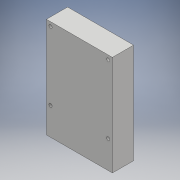
# Autodesk Inventor part: RaspberryPi_Placeholder
Saved by Autodesk Inventor 2017 (Build 210142000, 142)
## iProperties
Created: 2017-02-02
Part Number: RaspberryPi_Placeholder
Material: Generic
Document SubType Name: Modeling
Designer: Alexander Miller
Density: 1 g/cm^3
Appearance: Default
Author: Alexander Miller
Autodesk Inventor part; units mm, degrees
ref_plane "YZ Plane" through (0, 0, 0) normal (1, 0, 0) x (0, 1, 0)
ref_plane "XZ Plane" through (0, 0, 0) normal (0, 1, 0) x (-1, 0, 0)
ref_plane "XY Plane" through (0, 0, 0) normal (0, 0, 1) x (1, 0, 0)
sketch "Sketch1" plane through (0, 0, 0) normal (0, 1, 0) x (-1, 0, 0)
  line L0 (-28, 42.5) -> (28, 42.5)
  line L1 (28, 42.5) -> (28, -42.5)
  line L2 (28, -42.5) -> (-28, -42.5)
  line L3 (-28, -42.5) -> (-28, 42.5)
  point P0 (0, 0)
  point P1 (28, 0)
  point P2 (0, 42.5)
  dimension "d0" = 85
  dimension "d1" = 56
  constraints: 8 end point, 2 midpoint, 2 parallel, 1 horizontal, 1 horizontal alignment, 1 perpendicular, 1 vertical alignment
  measures "d0" distance of L0.end L1.end
  measures "d1" distance of L0.start L0.end
extrude "Extrusion1" add sketch "Sketch1" along normal blind 18
sketch "Sketch2" plane through (0, 18, 0) normal (0, 1, 0) x (1, 0, 0)
  circle A0 centre (-24.5, -39) radius 1.375
  circle A1 centre (24.5, -39) radius 1.375
  circle A2 centre (24.5, 19) radius 1.375
  circle A3 centre (-24.5, 19) radius 1.375
  line L0 (-28, 42.5) -> (-28, -42.5) projected
  line L1 (28, 42.5) -> (28, -42.5) projected
  line L2 (-28, -42.5) -> (28, -42.5) projected
  point P0 (0, 0)
  dimension "d4" = 3.5
  dimension "d5" = 3.5
  dimension "d6" = 58
  dimension "d7" = 2.75
  dimension "d8" = 3.5
  constraints: 4 centre point, 3 equal radius, 2 horizontal alignment, 2 vertical alignment
  measures "d4" distance from line of A0.centre L0
  measures "d5" distance from line of L1 A1.centre
  measures "d6" distance of A3.centre A0.centre
  measures "d7" diameter of A0
  measures "d8" distance from line of A1.centre L2
extrude "Extrusion2" cut sketch "Sketch2" against normal through all
equation "\"d5\" = d4"
equation "\"d8\" = d4"
body "Solid1"
